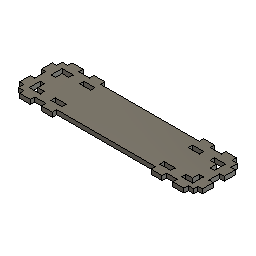
Rectangle_v1 (Autodesk Fusion 360 design; units mm, degrees)
Autodesk Fusion 360 part; units mm, degrees
sketch "Sketch1" plane through (0, 0, 0) normal (0, 1, 0) x (1, 0, 0)
  line L0 (0, 0) -> (120, 0)
  line L1 (120, 0) -> (120, -30)
  line L2 (120, -30) -> (0, -30)
  line L3 (0, -30) -> (0, 0)
  dimension "d3" = 120
  dimension "d4" = 30
  constraint horizontal L0
  constraint vertical L1
  constraint horizontal L2
  constraint vertical L3
  constraint coincident L0.start L3.end
  measures "d3" distance of L0.start L0.end
  measures "d4" distance of L0.start L2.end
extrude "Extrude1" add sketch "Sketch1" along normal blind 3
sketch "Sketch3" plane through (0, 0, 0) normal (0, 1, 0) x (1, 0, 0)
  line L0 (120, -30) -> (0, -30)
  line L1 (0, -30) -> (0, 0)
  line L2 (0, 0) -> (120, 0)
  line L3 (120, 0) -> (120, -30)
  line L4 (0, -26.25) -> (-3, -26.25)
  line L5 (-3, -26.25) -> (-3, -18.75)
  line L6 (-3, -18.75) -> (0, -18.75)
  line L7 (0, -18.75) -> (0, -26.25)
  line L8 (0, -11.25) -> (-3, -11.25)
  line L9 (-3, -11.25) -> (-3, -3.75)
  line L10 (-3, -3.75) -> (0, -3.75)
  line L11 (0, -3.75) -> (0, -11.25)
  line L12 (3.75, 0) -> (11.25, 0)
  line L13 (11.25, 0) -> (11.25, 3)
  line L14 (11.25, 3) -> (3.75, 3)
  line L15 (3.75, 3) -> (3.75, 0)
  line L16 (18.75, 0) -> (26.25, 0)
  line L17 (26.25, 0) -> (26.25, 3)
  line L18 (26.25, 3) -> (18.75, 3)
  line L19 (18.75, 3) -> (18.75, 0)
  line L20 (116.25, 0) -> (108.75, 0)
  line L21 (108.75, 0) -> (108.75, 3)
  line L22 (108.75, 3) -> (116.25, 3)
  line L23 (116.25, 3) -> (116.25, 0)
  line L24 (101.25, 0) -> (93.75, 0)
  line L25 (93.75, 0) -> (93.75, 3)
  line L26 (93.75, 3) -> (101.25, 3)
  line L27 (101.25, 3) -> (101.25, 0)
  line L28 (120, -4.6509) -> (123, -4.6509)
  line L29 (123, -4.6509) -> (123, -12.1509)
  line L30 (123, -12.1509) -> (120, -12.1509)
  line L31 (120, -12.1509) -> (120, -4.6509)
  line L32 (120, -19.6509) -> (123, -19.6509)
  line L33 (123, -19.6509) -> (123, -27.1509)
  line L34 (123, -27.1509) -> (120, -27.1509)
  line L35 (120, -27.1509) -> (120, -19.6509)
  line L36 (116.25, -30) -> (108.75, -30)
  line L37 (108.75, -30) -> (108.75, -33)
  line L38 (108.75, -33) -> (116.25, -33)
  line L39 (116.25, -33) -> (116.25, -30)
  line L40 (101.25, -30) -> (93.75, -30)
  line L41 (93.75, -30) -> (93.75, -33)
  line L42 (93.75, -33) -> (101.25, -33)
  line L43 (101.25, -33) -> (101.25, -30)
  line L44 (26.25, -30) -> (18.75, -30)
  line L45 (18.75, -30) -> (18.75, -33)
  line L46 (18.75, -33) -> (26.25, -33)
  line L47 (26.25, -33) -> (26.25, -30)
  line L48 (11.25, -30) -> (3.75, -30)
  line L49 (3.75, -30) -> (3.75, -33)
  line L50 (3.75, -33) -> (11.25, -33)
  line L51 (11.25, -33) -> (11.25, -30)
  line L52 (3.75, 3) -> (0, 3) construction
  line L53 (11.25, 3) -> (18.75, 3) construction
  line L54 (101.25, 3) -> (108.75, 3) construction
  line L55 (116.25, 3) -> (120, 3) construction
  line L56 (120, 0) -> (120, -4.6509) construction
  line L57 (123, -12.1509) -> (123, -19.6509) construction
  line L58 (108.75, -33) -> (101.25, -33) construction
  line L59 (120, -30) -> (116.25, -30) construction
  dimension "d10" = 3
  dimension "d11" = 7.5
  dimension "d13" = 3
  dimension "d14" = 3.75
  dimension "d15" = 3.75
  dimension "d16" = 7.5
  dimension "d17" = 7.5
  dimension "d18" = 3.75
  dimension "d19" = 3.75
  dimension "d20" = 7.5
  dimension "d21" = 7.5
  dimension "d22" = 3.75
  dimension "d23" = 7.5
  dimension "d24" = 7.5
  dimension "d25" = 3.75
  constraint horizontal L4
  constraint vertical L5
  constraint horizontal L6
  constraint vertical L7
  constraint coincident L1 L4.start
  constraint horizontal L8
  constraint vertical L9
  constraint horizontal L10
  constraint vertical L11
  constraint coincident L1 L8.start
  constraint horizontal L12
  constraint vertical L13
  constraint horizontal L14
  constraint vertical L15
  constraint coincident L2 L12.start
  constraint horizontal L16
  constraint vertical L17
  constraint horizontal L18
  constraint vertical L19
  constraint coincident L2 L16.start
  constraint horizontal L20
  constraint vertical L21
  constraint horizontal L22
  constraint vertical L23
  constraint coincident L2 L20.start
  constraint horizontal L24
  constraint vertical L25
  constraint horizontal L26
  constraint vertical L27
  constraint coincident L2 L24.start
  constraint horizontal L28
  constraint vertical L29
  constraint horizontal L30
  constraint vertical L31
  constraint coincident L3 L28.start
  constraint horizontal L32
  constraint vertical L33
  constraint horizontal L34
  constraint vertical L35
  constraint coincident L3 L32.start
  constraint horizontal L36
  constraint vertical L37
  constraint horizontal L38
  constraint vertical L39
  constraint coincident L0 L36.start
  constraint horizontal L40
  constraint vertical L41
  constraint horizontal L42
  constraint vertical L43
  constraint coincident L0 L40.start
  constraint horizontal L44
  constraint vertical L45
  constraint horizontal L46
  constraint vertical L47
  constraint coincident L0 L44.start
  constraint horizontal L48
  constraint vertical L49
  constraint horizontal L50
  constraint vertical L51
  constraint coincident L0 L48.start
  constraint equal L4 L8
  constraint equal L45 L51
  constraint equal L41 L47
  constraint equal L37 L41
  constraint equal L34 L39
  constraint equal L30 L32
  constraint equal L23 L28
  constraint equal L21 L27
  constraint equal L17 L25
  constraint equal L13 L19
  constraint equal L5 L9
  constraint equal L5 L50
  constraint equal L46 L50
  constraint equal L42 L46
  constraint equal L38 L42
  constraint equal L33 L38
  constraint equal L29 L33
  constraint equal L22 L29
  constraint equal L22 L26
  constraint equal L18 L26
  constraint equal L14 L18
  constraint perpendicular L15 L52
  constraint perpendicular L31 L55
  constraint coincident L2.end L3.start
  constraint coincident L0.start L3.end
  constraint coincident L55.end L56
  constraint coincident L1 L52.end
  measures "d10" distance of L4.start L4.end
  measures "d11" distance of L8.end L9.end
  measures "d13" distance of L48.end L49.end
  measures "d14" distance of L0.end L4
  measures "d15" distance of L0.end L49
  measures "d16" distance of L45 L51
  measures "d17" distance of L6 L8
  measures "d18" distance of L1.end L10
  measures "d19" distance of L36.start L0.start
  measures "d20" distance of L37.end L42.end
  measures "d21" distance of L29.end L32.end
  measures "d22" distance of L22.end L55.end
  measures "d23" distance of L21.end L26.end
  measures "d24" distance of L13.end L18.end
  measures "d25" distance of L14.end L52.end
extrude "Extrude2" add sketch "Sketch3" along normal blind 3 contours L0 L36 L37 L38 L39 | L3 L32 L33 L34 L35 | L0 L40 L41 L42 L43 | L3 L28 L29 L30 L31 | L0 L44 L45 L46 L47 | L2 L20 L21 L22 L23 | L0 L48 L49 L50 L51 | L2 L24 L25 L26 L27 | L1 L4 L5 L6 L7 | L2 L16 L17 L18 L19 | L1 L8 L9 L10 L11 | L2 L12 L13 L14 L15
sketch "Sketch4" plane through (0, 0, 0) normal (0, 1, 0) x (1, 0, 0)
  line L0 (120, -30) -> (116.25, -30)
  line L1 (116.25, -30) -> (116.25, -33)
  line L2 (116.25, -33) -> (108.75, -33)
  line L3 (108.75, -33) -> (108.75, -30)
  line L4 (108.75, -30) -> (101.25, -30)
  line L5 (101.25, -30) -> (101.25, -33)
  line L6 (101.25, -33) -> (93.75, -33)
  line L7 (93.75, -33) -> (93.75, -30)
  line L8 (93.75, -30) -> (26.25, -30)
  line L9 (26.25, -30) -> (26.25, -33)
  line L10 (26.25, -33) -> (18.75, -33)
  line L11 (18.75, -33) -> (18.75, -30)
  line L12 (18.75, -30) -> (11.25, -30)
  line L13 (11.25, -30) -> (11.25, -33)
  line L14 (11.25, -33) -> (3.75, -33)
  line L15 (3.75, -33) -> (3.75, -30)
  line L16 (3.75, -30) -> (0, -30)
  line L17 (0, -30) -> (0, -26.25)
  line L18 (0, -26.25) -> (-3, -26.25)
  line L19 (-3, -26.25) -> (-3, -18.75)
  line L20 (-3, -18.75) -> (0, -18.75)
  line L21 (0, -18.75) -> (0, -11.25)
  line L22 (0, -11.25) -> (-3, -11.25)
  line L23 (-3, -11.25) -> (-3, -3.75)
  line L24 (-3, -3.75) -> (0, -3.75)
  line L25 (0, -3.75) -> (0, 0)
  line L26 (0, 0) -> (3.75, 0)
  line L27 (3.75, 0) -> (3.75, 3)
  line L28 (3.75, 3) -> (11.25, 3)
  line L29 (11.25, 3) -> (11.25, 0)
  line L30 (11.25, 0) -> (18.75, 0)
  line L31 (18.75, 0) -> (18.75, 3)
  line L32 (18.75, 3) -> (26.25, 3)
  line L33 (26.25, 3) -> (26.25, 0)
  line L34 (26.25, 0) -> (93.75, 0)
  line L35 (93.75, 0) -> (93.75, 3)
  line L36 (93.75, 3) -> (101.25, 3)
  line L37 (101.25, 3) -> (101.25, 0)
  line L38 (101.25, 0) -> (108.75, 0)
  line L39 (108.75, 0) -> (108.75, 3)
  line L40 (108.75, 3) -> (116.25, 3)
  line L41 (116.25, 3) -> (116.25, 0)
  line L42 (116.25, 0) -> (120, 0)
  line L43 (120, 0) -> (120, -4.6509)
  line L44 (120, -4.6509) -> (123, -4.6509)
  line L45 (123, -4.6509) -> (123, -12.1509)
  line L46 (123, -12.1509) -> (120, -12.1509)
  line L47 (120, -12.1509) -> (120, -19.6509)
  line L48 (120, -19.6509) -> (123, -19.6509)
  line L49 (123, -19.6509) -> (123, -27.1509)
  line L50 (123, -27.1509) -> (120, -27.1509)
  line L51 (120, -27.1509) -> (120, -30)
  line L52 (116.25, 0) -> (116.25, -30) construction
  line L53 (120, -27.1509) -> (0, -26.25) construction
  line L54 (0, -18.75) -> (120, -19.6509) construction
  line L55 (120, -12.1509) -> (0, -11.25) construction
  line L56 (0, -3.75) -> (120, -4.6509) construction
  line L57 (108.75, 0) -> (108.75, -30) construction
  line L58 (101.25, -30) -> (101.25, 0) construction
  line L59 (93.75, 0) -> (93.75, -30) construction
  line L60 (26.25, -30) -> (26.25, 0) construction
  line L61 (18.75, 0) -> (18.75, -30) construction
  line L62 (11.25, -30) -> (11.25, 0) construction
  line L63 (3.75, 0) -> (3.75, -30) construction
  line L64 (116.25, -4.6227) -> (113.25, -4.6227)
  line L65 (113.25, -4.6227) -> (113.25, -12.1002)
  line L66 (113.25, -12.1002) -> (116.25, -12.1002)
  line L67 (116.25, -12.1002) -> (116.25, -4.6227)
  line L68 (108.75, -4.5664) -> (116.25, -4.5664)
  line L69 (116.25, -4.5664) -> (116.25, -7.5664)
  line L70 (116.25, -7.5664) -> (108.75, -7.5664)
  line L71 (108.75, -7.5664) -> (108.75, -4.5664)
  line L72 (101.25, -4.5101) -> (93.75, -4.5101)
  line L73 (93.75, -4.5101) -> (93.75, -7.5101)
  line L74 (93.75, -7.5101) -> (101.25, -7.5101)
  line L75 (101.25, -7.5101) -> (101.25, -4.5101)
  line L76 (116.25, -19.6227) -> (113.25, -19.6227)
  line L77 (113.25, -19.6227) -> (113.25, -27.1002)
  line L78 (113.25, -27.1002) -> (116.25, -27.1002)
  line L79 (116.25, -27.1002) -> (116.25, -19.6227)
  line L80 (108.75, -27.0664) -> (116.25, -27.0664)
  line L81 (116.25, -27.0664) -> (116.25, -24.0664)
  line L82 (116.25, -24.0664) -> (108.75, -24.0664)
  line L83 (108.75, -24.0664) -> (108.75, -27.0664)
  line L84 (101.25, -27.0101) -> (93.75, -27.0101)
  line L85 (93.75, -27.0101) -> (93.75, -24.0101)
  line L86 (93.75, -24.0101) -> (101.25, -24.0101)
  line L87 (101.25, -24.0101) -> (101.25, -27.0101)
  line L88 (26.25, -26.4471) -> (18.75, -26.4471)
  line L89 (18.75, -26.4471) -> (18.75, -23.4471)
  line L90 (18.75, -23.4471) -> (26.25, -23.4471)
  line L91 (26.25, -23.4471) -> (26.25, -26.4471)
  line L92 (11.25, -26.3345) -> (3.75, -26.3345)
  line L93 (3.75, -26.3345) -> (3.75, -23.3345)
  line L94 (3.75, -23.3345) -> (11.25, -23.3345)
  line L95 (11.25, -23.3345) -> (11.25, -26.3345)
  line L96 (3.75, -18.7782) -> (6.75, -18.7782)
  line L97 (6.75, -18.7782) -> (6.75, -26.3345)
  line L98 (6.75, -26.3345) -> (3.75, -26.3345)
  line L99 (3.75, -26.3345) -> (3.75, -18.7782)
  line L100 (3.75, -11.2782) -> (6.75, -11.2782)
  line L101 (6.75, -11.2782) -> (6.75, -3.8007)
  line L102 (6.75, -3.8007) -> (3.75, -3.8007)
  line L103 (3.75, -3.8007) -> (3.75, -11.2782)
  line L104 (3.75, -3.8007) -> (11.25, -3.8007)
  line L105 (11.25, -3.8007) -> (11.25, -6.8007)
  line L106 (11.25, -6.8007) -> (3.75, -6.8007)
  line L107 (3.75, -6.8007) -> (3.75, -3.8007)
  line L108 (18.75, -3.8908) -> (26.25, -3.8908)
  line L109 (26.25, -3.8908) -> (26.25, -6.8908)
  line L110 (26.25, -6.8908) -> (18.75, -6.8908)
  line L111 (18.75, -6.8908) -> (18.75, -3.8908)
  dimension "d28" = 3
  dimension "d29" = 3
  dimension "d30" = 3
  dimension "d31" = 3
  dimension "d32" = 3
  dimension "d33" = 3
  constraint coincident L41.end L42.start
  constraint coincident L0.end L1.start
  constraint coincident L50.end L51.start
  constraint coincident L17.end L18.start
  constraint coincident L20.end L21.start
  constraint coincident L47.end L48.start
  constraint coincident L46.end L47.start
  constraint coincident L21.end L22.start
  constraint coincident L24.end L25.start
  constraint coincident L43.end L44.start
  constraint coincident L38.end L39.start
  constraint coincident L3.end L4.start
  constraint coincident L4.end L5.start
  constraint coincident L37.end L38.start
  constraint coincident L34.end L35.start
  constraint coincident L7.end L8.start
  constraint coincident L8.end L9.start
  constraint coincident L33.end L34.start
  constraint coincident L30.end L31.start
  constraint coincident L11.end L12.start
  constraint coincident L12.end L13.start
  constraint coincident L29.end L30.start
  constraint coincident L26.end L27.start
  constraint coincident L15.end L16.start
  constraint horizontal L64
  constraint vertical L65
  constraint horizontal L66
  constraint vertical L67
  constraint coincident L55 L65.end
  constraint coincident L52 L64.start
  constraint coincident L56 L64.start
  constraint horizontal L68
  constraint vertical L69
  constraint horizontal L70
  constraint vertical L71
  constraint coincident L52 L69.end
  constraint coincident L57 L68.start
  constraint coincident L56 L68.start
  constraint horizontal L72
  constraint vertical L73
  constraint horizontal L74
  constraint vertical L75
  constraint coincident L59 L73.end
  constraint coincident L58 L72.start
  constraint coincident L56 L72.start
  constraint horizontal L76
  constraint vertical L77
  constraint horizontal L78
  constraint vertical L79
  constraint coincident L53 L77.end
  constraint coincident L52 L76.start
  constraint coincident L54 L76.start
  constraint horizontal L80
  constraint vertical L81
  constraint horizontal L82
  constraint vertical L83
  constraint coincident L79 L81.end
  constraint coincident L53 L80.start
  constraint coincident L57 L80.start
  constraint horizontal L84
  constraint vertical L85
  constraint horizontal L86
  constraint vertical L87
  constraint coincident L59 L85.end
  constraint coincident L58 L84.start
  constraint coincident L53 L84.start
  constraint horizontal L88
  constraint vertical L89
  constraint horizontal L90
  constraint vertical L91
  constraint coincident L61 L89.end
  constraint coincident L60 L88.start
  constraint coincident L53 L88.start
  constraint horizontal L92
  constraint vertical L93
  constraint horizontal L94
  constraint vertical L95
  constraint coincident L63 L93.end
  constraint coincident L53 L92.start
  constraint coincident L62 L92.start
  constraint horizontal L96
  constraint vertical L97
  constraint horizontal L98
  constraint vertical L99
  constraint coincident L63 L96.start
  constraint coincident L54 L96.start
  constraint horizontal L100
  constraint vertical L101
  constraint horizontal L102
  constraint vertical L103
  constraint coincident L56 L101.end
  constraint coincident L63 L100.start
  constraint coincident L55 L100.start
  constraint horizontal L104
  constraint vertical L105
  constraint horizontal L106
  constraint vertical L107
  constraint coincident L62 L105.end
  constraint horizontal L108
  constraint vertical L109
  constraint horizontal L110
  constraint vertical L111
  constraint coincident L60 L109.end
  constraint coincident L61 L108.start
  constraint coincident L56 L108.start
  constraint equal L71 L75
  constraint equal L73 L109
  constraint equal L105 L111
  constraint equal L100 L107
  constraint coincident L92.end L98
  constraint equal L89 L95
  constraint equal L83 L87
  measures "d28" distance of L63 L101
  measures "d29" distance of L97 L99
  measures "d30" distance of L52 L77
  measures "d31" distance of L65 L67
  measures "d32" distance of L92.start L94
  measures "d33" distance of L84.end L86
extrude "Extrude3" cut sketch "Sketch4" along normal up to surface (3 mm away) contours L64 L65 L67 L69 L70 | L64 L65 L68 L69 L70 L71 | L65 L66 L67 L70 | L72 L73 L74 L75 | L76 L77 L79 L82 | L77 L79 L80 L81 L82 | L77 L80 L82 L83 | L84 L85 L86 L87 | L88 L89 L90 L91 | L92 L94 L95 L97 | L92 L93 L94 L97 L98 L99 | L94 L96 L97 L99 | L100 L101 L103 L106 | L101 L102 L103 L104 L106 L107 | L101 L104 L105 L106 | L108 L109 L110 L111
equation "main_length = 120 mm"
equation "main_width = 30 mm"
equation "d3 = main_length"
equation "d4 = main_width"
equation "material_thickness = 3 mm"
equation "d6 = material_thickness"
equation "fit_length = 7.5 mm"
equation "fit_spacing = 7.5 mm"
equation "d10 = material_thickness"
equation "d11 = fit_length"
equation "d13 = material_thickness"
equation "d14 = fit_spacing / 2"
equation "d15 = fit_spacing / 2"
equation "d16 = fit_spacing"
equation "d17 = fit_spacing"
equation "d19 = fit_spacing / 2"
equation "d20 = fit_spacing"
equation "d21 = fit_spacing"
equation "d22 = fit_spacing / 2"
equation "d23 = fit_spacing"
equation "d24 = fit_spacing"
equation "d25 = fit_spacing / 2"
equation "d28 = material_thickness"
equation "d29 = material_thickness"
equation "d30 = material_thickness"
equation "d31 = material_thickness"
equation "d32 = material_thickness"
equation "d33 = material_thickness"
